Autodesk Fusion 360 part; units mm, degrees
(part 14 of 19)
  spline S154 degree 3 poles (24.0633, 11.8257) (24.3884, 11.9073) (24.7337, 11.9631) (25.4345, 12.0396) (25.8145, 12.0581) (26.1868, 12.059) knots -0.210627 -0.210627 -0.210627 -0.210627 -0.111696 -0.111696 0 0 0 0
  spline S155 degree 3 poles (23.9494, 11.8782) (23.9537, 11.8696) (23.9592, 11.8616) (23.9723, 11.8475) (23.9799, 11.8414) (23.9994, 11.8299) (24.0118, 11.8255) (24.0376, 11.8218) (24.0507, 11.8225) (24.0633, 11.8257) knots -0.013599 -0.013599 -0.013599 -0.013599 -0.010706 -0.010706 -0.007813 -0.007813 -0.003906 -0.003906 0 0 0 0
  arc A79 (23.9494, 11.8782) -> (23.6868, 12.3936) centre (0, 0) ccw
  spline S156 degree 3 poles (23.7112, 12.5167) (23.7038, 12.5105) (23.6974, 12.5033) (23.6867, 12.4872) (23.6826, 12.4784) (23.6759, 12.4568) (23.6746, 12.4437) (23.677, 12.4178) (23.6807, 12.4051) (23.6868, 12.3936) knots -0.013599 -0.013599 -0.013599 -0.013599 -0.010706 -0.010706 -0.007813 -0.007813 -0.003906 -0.003906 0 0 0 0
  spline S157 degree 3 poles (25.1482, 14.0975) (24.9286, 13.7968) (24.6903, 13.5003) (24.2164, 12.9783) (23.9684, 12.7317) (23.7112, 12.5167) knots -0.220678 -0.220678 -0.220678 -0.220678 -0.107909 -0.107909 -0.008028 -0.008028 -0.008028 -0.008028
  arc A80 (25.1482, 14.0975) -> (24.7828, 14.7302) centre (0, 0) ccw
  spline S158 degree 3 poles (22.6954, 14.2762) (23.0102, 14.3914) (23.3477, 14.4829) (24.0367, 14.6323) (24.4127, 14.6904) (24.7828, 14.7302) knots -0.210627 -0.210627 -0.210627 -0.210627 -0.111696 -0.111696 0 0 0 0
  spline S159 degree 3 poles (22.5766, 14.3165) (22.5817, 14.3084) (22.588, 14.301) (22.6026, 14.2884) (22.6107, 14.2831) (22.6313, 14.2737) (22.6441, 14.2707) (22.6702, 14.2697) (22.6831, 14.2717) (22.6954, 14.2762) knots -0.013599 -0.013599 -0.013599 -0.013599 -0.010706 -0.010706 -0.007813 -0.007813 -0.003906 -0.003906 0 0 0 0
  arc A81 (22.5766, 14.3165) -> (22.2615, 14.8017) centre (0, 0) ccw
  spline S160 degree 3 poles (22.273, 14.9266) (22.2663, 14.9197) (22.2606, 14.9118) (22.2517, 14.8947) (22.2485, 14.8856) (22.2441, 14.8633) (22.2442, 14.8502) (22.2493, 14.8246) (22.2543, 14.8125) (22.2615, 14.8017) knots -0.013599 -0.013599 -0.013599 -0.013599 -0.010706 -0.010706 -0.007813 -0.007813 -0.003906 -0.003906 0 0 0 0
  spline S161 degree 3 poles (23.5368, 16.6489) (23.3499, 16.327) (23.1439, 16.0071) (22.7272, 15.4385) (22.5063, 15.1674) (22.273, 14.9266) knots -0.220678 -0.220678 -0.220678 -0.220678 -0.107909 -0.107909 -0.008028 -0.008028 -0.008028 -0.008028
  arc A82 (23.5368, 16.6489) -> (23.1074, 17.24) centre (0, 0) ccw
  spline S162 degree 3 poles (21.0788, 16.5703) (21.3798, 16.7177) (21.7059, 16.8441) (22.3755, 17.0646) (22.7434, 17.1617) (23.1074, 17.24) knots -0.210627 -0.210627 -0.210627 -0.210627 -0.111696 -0.111696 0 0 0 0
  spline S163 degree 3 poles (20.9564, 16.598) (20.9624, 16.5904) (20.9694, 16.5838) (20.9852, 16.5727) (20.9939, 16.5683) (21.0154, 16.5611) (21.0284, 16.5594) (21.0544, 16.5612) (21.0671, 16.5645) (21.0788, 16.5703) knots -0.013599 -0.013599 -0.013599 -0.013599 -0.010706 -0.010706 -0.007813 -0.007813 -0.003906 -0.003906 0 0 0 0
  arc A83 (20.9564, 16.598) -> (20.5924, 17.0475) centre (0, 0) ccw
  spline S164 degree 3 poles (20.5907, 17.173) (20.5848, 17.1654) (20.5799, 17.157) (20.5728, 17.1391) (20.5706, 17.1296) (20.5686, 17.1071) (20.5701, 17.094) (20.5778, 17.0691) (20.5841, 17.0576) (20.5924, 17.0475) knots -0.013599 -0.013599 -0.013599 -0.013599 -0.010706 -0.010706 -0.007813 -0.007813 -0.003906 -0.003906 0 0 0 0
  spline S165 degree 3 poles (21.6676, 19.018) (21.5153, 18.6782) (21.3439, 18.3387) (20.9889, 17.7295) (20.7975, 17.4368) (20.5907, 17.173) knots -0.220678 -0.220678 -0.220678 -0.220678 -0.107909 -0.107909 -0.008028 -0.008028 -0.008028 -0.008028
  arc A84 (21.6676, 19.018) -> (21.1787, 19.561) centre (0, 0) ccw
  spline S166 degree 3 poles (19.2312, 18.6828) (19.5152, 18.861) (19.8263, 19.0207) (20.4692, 19.31) (20.8249, 19.445) (21.1787, 19.561) knots -0.210627 -0.210627 -0.210627 -0.210627 -0.111696 -0.111696 0 0 0 0
  spline S167 degree 3 poles (19.1066, 18.6976) (19.1134, 18.6907) (19.1211, 18.6848) (19.1379, 18.6755) (19.147, 18.672) (19.1691, 18.6671) (19.1823, 18.6668) (19.2079, 18.6712) (19.2202, 18.6759) (19.2312, 18.6828) knots -0.013599 -0.013599 -0.013599 -0.013599 -0.010706 -0.010706 -0.007813 -0.007813 -0.003906 -0.003906 0 0 0 0
  arc A85 (19.1066, 18.6976) -> (18.6976, 19.1066) centre (0, 0) ccw
  spline S168 degree 3 poles (18.6828, 19.2312) (18.6777, 19.2231) (18.6738, 19.2142) (18.6686, 19.1956) (18.6674, 19.186) (18.6678, 19.1633) (18.6706, 19.1505) (18.6809, 19.1266) (18.6883, 19.1157) (18.6976, 19.1066) knots -0.013599 -0.013599 -0.013599 -0.013599 -0.010706 -0.010706 -0.007813 -0.007813 -0.003906 -0.003906 0 0 0 0
  spline S169 degree 3 poles (19.561, 21.1787) (19.445, 20.8249) (19.31, 20.4692) (19.0207, 19.8263) (18.861, 19.5152) (18.6828, 19.2312) knots -0.220678 -0.220678 -0.220678 -0.220678 -0.107909 -0.107909 -0.008028 -0.008028 -0.008028 -0.008028
  arc A86 (19.561, 21.1787) -> (19.018, 21.6676) centre (0, 0) ccw
  spline S170 degree 3 poles (17.173, 20.5907) (17.4368, 20.7975) (17.7295, 20.9889) (18.3387, 21.3439) (18.6782, 21.5153) (19.018, 21.6676) knots -0.210627 -0.210627 -0.210627 -0.210627 -0.111696 -0.111696 0 0 0 0
  spline S171 degree 3 poles (17.0475, 20.5924) (17.055, 20.5862) (17.0632, 20.5812) (17.081, 20.5736) (17.0904, 20.5711) (17.1129, 20.5686) (17.126, 20.5696) (17.151, 20.5767) (17.1628, 20.5827) (17.173, 20.5907) knots -0.013599 -0.013599 -0.013599 -0.013599 -0.010706 -0.010706 -0.007813 -0.007813 -0.003906 -0.003906 0 0 0 0
  arc A87 (17.0475, 20.5924) -> (16.598, 20.9564) centre (0, 0) ccw
  spline S172 degree 3 poles (16.5703, 21.0788) (16.566, 21.0701) (16.5631, 21.0609) (16.5599, 21.0419) (16.5597, 21.0322) (16.5624, 21.0097) (16.5665, 20.9972) (16.5793, 20.9745) (16.5878, 20.9645) (16.598, 20.9564) knots -0.013599 -0.013599 -0.013599 -0.013599 -0.010706 -0.010706 -0.007813 -0.007813 -0.003906 -0.003906 0 0 0 0
  spline S173 degree 3 poles (17.24, 23.1074) (17.1617, 22.7434) (17.0646, 22.3755) (16.8441, 21.7059) (16.7177, 21.3798) (16.5703, 21.0788) knots -0.220678 -0.220678 -0.220678 -0.220678 -0.107909 -0.107909 -0.008028 -0.008028 -0.008028 -0.008028
  arc A88 (17.24, 23.1074) -> (16.6489, 23.5368) centre (0, 0) ccw
  spline S174 degree 3 poles (14.9266, 22.273) (15.1674, 22.5063) (15.4385, 22.7272) (16.0071, 23.1439) (16.327, 23.3499) (16.6489, 23.5368) knots -0.210627 -0.210627 -0.210627 -0.210627 -0.111696 -0.111696 0 0 0 0
  spline S175 degree 3 poles (14.8017, 22.2615) (14.8097, 22.2562) (14.8184, 22.252) (14.8369, 22.2464) (14.8465, 22.2449) (14.8691, 22.2447) (14.882, 22.2471) (14.9062, 22.2568) (14.9173, 22.2639) (14.9266, 22.273) knots -0.013599 -0.013599 -0.013599 -0.013599 -0.010706 -0.010706 -0.007813 -0.007813 -0.003906 -0.003906 0 0 0 0
  arc A89 (14.8017, 22.2615) -> (14.3165, 22.5766) centre (0, 0) ccw
  spline S176 degree 3 poles (14.2762, 22.6954) (14.2729, 22.6863) (14.2709, 22.6768) (14.2697, 22.6576) (14.2705, 22.6479) (14.2756, 22.6258) (14.2809, 22.6138) (14.296, 22.5926) (14.3055, 22.5835) (14.3165, 22.5766) knots -0.013599 -0.013599 -0.013599 -0.013599 -0.010706 -0.010706 -0.007813 -0.007813 -0.003906 -0.003906 0 0 0 0
  spline S177 degree 3 poles (14.7302, 24.7828) (14.6904, 24.4127) (14.6323, 24.0367) (14.4829, 23.3477) (14.3914, 23.0102) (14.2762, 22.6954) knots -0.220678 -0.220678 -0.220678 -0.220678 -0.107909 -0.107909 -0.008028 -0.008028 -0.008028 -0.008028
  arc A90 (14.7302, 24.7828) -> (14.0975, 25.1482) centre (0, 0) ccw
  spline S178 degree 3 poles (12.5167, 23.7112) (12.7317, 23.9684) (12.9783, 24.2164) (13.5003, 24.6903) (13.7968, 24.9286) (14.0975, 25.1482) knots -0.210627 -0.210627 -0.210627 -0.210627 -0.111696 -0.111696 0 0 0 0
  spline S179 degree 3 poles (12.3936, 23.6868) (12.4022, 23.6823) (12.4113, 23.6791) (12.4302, 23.6754) (12.4399, 23.6749) (12.4625, 23.6771) (12.4751, 23.6808) (12.4981, 23.693) (12.5083, 23.7012) (12.5167, 23.7112) knots -0.013599 -0.013599 -0.013599 -0.013599 -0.010706 -0.010706 -0.007813 -0.007813 -0.003906 -0.003906 0 0 0 0
  arc A91 (12.3936, 23.6868) -> (11.8782, 23.9494) centre (0, 0) ccw
  spline S180 degree 3 poles (11.8257, 24.0633) (11.8233, 24.054) (11.8223, 24.0443) (11.8231, 24.025) (11.8249, 24.0155) (11.8323, 23.9941) (11.8389, 23.9827) (11.8561, 23.9632) (11.8665, 23.9552) (11.8782, 23.9494) knots -0.013599 -0.013599 -0.013599 -0.013599 -0.010706 -0.010706 -0.007813 -0.007813 -0.003906 -0.003906 0 0 0 0
  spline S181 degree 3 poles (12.059, 26.1868) (12.0581, 25.8145) (12.0396, 25.4345) (11.9631, 24.7337) (11.9073, 24.3884) (11.8257, 24.0633) knots -0.220678 -0.220678 -0.220678 -0.220678 -0.107909 -0.107909 -0.008028 -0.008028 -0.008028 -0.008028
  arc A92 (12.059, 26.1868) -> (11.3915, 26.484) centre (0, 0) ccw
  spline S182 degree 3 poles (9.9696, 24.8897) (10.1566, 25.1679) (10.3759, 25.4404) (10.8455, 25.9662) (11.1155, 26.2342) (11.3915, 26.484) knots -0.210627 -0.210627 -0.210627 -0.210627 -0.111696 -0.111696 0 0 0 0
  spline S183 degree 3 poles (9.8498, 24.8525) (9.8587, 24.8489) (9.8682, 24.8467) (9.8874, 24.845) (9.8971, 24.8455) (9.9193, 24.85) (9.9314, 24.8551) (9.9531, 24.8696) (9.9624, 24.8789) (9.9696, 24.8897) knots -0.013599 -0.013599 -0.013599 -0.013599 -0.010706 -0.010706 -0.007813 -0.007813 -0.003906 -0.003906 0 0 0 0
  arc A93 (9.8498, 24.8525) -> (9.3097, 25.0598) centre (0, 0) ccw
  spline S184 degree 3 poles (9.2456, 25.1676) (9.2442, 25.1581) (9.2442, 25.1484) (9.2471, 25.1293) (9.2499, 25.12) (9.2594, 25.0995) (9.2672, 25.0888) (9.2863, 25.0712) (9.2975, 25.0643) (9.3097, 25.0598) knots -0.013599 -0.013599 -0.013599 -0.013599 -0.010706 -0.010706 -0.007813 -0.007813 -0.003906 -0.003906 0 0 0 0
  spline S185 degree 3 poles (9.2557, 27.3039) (9.2937, 26.9335) (9.315, 26.5537) (9.3122, 25.8487) (9.2928, 25.4995) (9.2456, 25.1676) knots -0.220678 -0.220678 -0.220678 -0.220678 -0.107909 -0.107909 -0.008028 -0.008028 -0.008028 -0.008028
  arc A94 (9.2557, 27.3039) -> (8.5608, 27.5296) centre (0, 0) ccw
  spline S186 degree 3 poles (7.3133, 25.7954) (7.4702, 26.0917) (7.6598, 26.3856) (8.0719, 26.9576) (8.3124, 27.2523) (8.5608, 27.5296) knots -0.210627 -0.210627 -0.210627 -0.210627 -0.111696 -0.111696 0 0 0 0
  spline S187 degree 3 poles (7.198, 25.7459) (7.2073, 25.7433) (7.2169, 25.7421) (7.2362, 25.7424) (7.2458, 25.7439) (7.2674, 25.7508) (7.2789, 25.757) (7.2989, 25.7737) (7.3072, 25.7839) (7.3133, 25.7954) knots -0.013599 -0.013599 -0.013599 -0.013599 -0.010706 -0.010706 -0.007813 -0.007813 -0.003906 -0.003906 0 0 0 0
  arc A95 (7.198, 25.7459) -> (6.6393, 25.8956) centre (0, 0) ccw
  spline S188 degree 3 poles (6.5642, 25.9962) (6.5638, 25.9865) (6.5649, 25.9769) (6.5697, 25.9582) (6.5734, 25.9493) (6.5851, 25.9298) (6.5939, 25.9201) (6.6148, 25.9045) (6.6267, 25.8989) (6.6393, 25.8956) knots -0.013599 -0.013599 -0.013599 -0.013599 -0.010706 -0.010706 -0.007813 -0.007813 -0.003906 -0.003906 0 0 0 0
  spline S189 degree 3 poles (6.351, 28.1218) (6.4275, 27.7574) (6.4884, 27.3819) (6.5592, 26.6805) (6.5765, 26.3312) (6.5642, 25.9962) knots -0.220678 -0.220678 -0.220678 -0.220678 -0.107909 -0.107909 -0.008028 -0.008028 -0.008028 -0.008028
  arc A96 (6.351, 28.1218) -> (5.6363, 28.2737) centre (0, 0) ccw
  spline S190 degree 3 poles (4.5769, 26.4186) (4.702, 26.7296) (4.8598, 27.0417) (5.2098, 27.6537) (5.4182, 27.9719) (5.6363, 28.2737) knots -0.210627 -0.210627 -0.210627 -0.210627 -0.111696 -0.111696 0 0 0 0
  spline S191 degree 3 poles (4.4674, 26.3573) (4.4769, 26.3557) (4.4866, 26.3554) (4.5058, 26.3578) (4.5151, 26.3603) (4.5359, 26.3693) (4.5467, 26.3768) (4.5649, 26.3955) (4.572, 26.4065) (4.5769, 26.4186) knots -0.013599 -0.013599 -0.013599 -0.013599 -0.010706 -0.010706 -0.007813 -0.007813 -0.003906 -0.003906 0 0 0 0
  arc A97 (4.4674, 26.3573) -> (3.8961, 26.4478) centre (0, 0) ccw
  spline S192 degree 3 poles (3.8109, 26.5399) (3.8115, 26.5303) (3.8136, 26.5208) (3.8203, 26.5027) (3.825, 26.4942) (3.8386, 26.4761) (3.8484, 26.4674) (3.8708, 26.4541) (3.8832, 26.4497) (3.8961, 26.4478) knots -0.013599 -0.013599 -0.013599 -0.013599 -0.010706 -0.010706 -0.007813 -0.007813 -0.003906 -0.003906 0 0 0 0
  spline S193 degree 3 poles (3.3766, 28.6316) (3.4908, 28.2772) (3.5906, 27.9101) (3.7344, 27.2199) (3.7881, 26.8744) (3.8109, 26.5399) knots -0.220678 -0.220678 -0.220678 -0.220678 -0.107909 -0.107909 -0.008028 -0.008028 -0.008028 -0.008028
  arc A98 (3.3766, 28.6316) -> (2.65, 28.708) centre (0, 0) ccw
  spline S194 degree 3 poles (1.7903, 26.7523) (1.8822, 27.0747) (2.0065, 27.4015) (2.2907, 28.0467) (2.4646, 28.385) (2.65, 28.708) knots -0.210627 -0.210627 -0.210627 -0.210627 -0.111696 -0.111696 0 0 0 0
  spline S195 degree 3 poles (1.6879, 26.6799) (1.6975, 26.6793) (1.7071, 26.68) (1.7259, 26.6844) (1.735, 26.6879) (1.7547, 26.699) (1.7647, 26.7076) (1.7808, 26.728) (1.7868, 26.7397) (1.7903, 26.7523) knots -0.013599 -0.013599 -0.013599 -0.013599 -0.010706 -0.010706 -0.007813 -0.007813 -0.003906 -0.003906 0 0 0 0
  arc A99 (1.6879, 26.6799) -> (1.1102, 26.7101) centre (0, 0) ccw
  spline S196 degree 3 poles (1.0158, 26.7929) (1.0175, 26.7834) (1.0205, 26.7741) (1.0291, 26.7569) (1.0346, 26.7489) (1.0501, 26.7323) (1.0607, 26.7246) (1.0844, 26.7138) (1.0972, 26.7107) (1.1102, 26.7101) knots -0.013599 -0.013599 -0.013599 -0.013599 -0.010706 -0.010706 -0.007813 -0.007813 -0.003906 -0.003906 0 0 0 0
  spline S197 degree 3 poles (0.3653, 28.8277) (0.5159, 28.4872) (0.6536, 28.1325) (0.8687, 27.4612) (0.9582, 27.1231) (1.0158, 26.7929) knots -0.220678 -0.220678 -0.220678 -0.220678 -0.107909 -0.107909 -0.008028 -0.008028 -0.008028 -0.008028
  arc A100 (0.3653, 28.8277) -> (-0.3653, 28.8277) centre (0, 0) ccw
  spline S198 degree 3 poles (-1.0158, 26.7929) (-0.9582, 27.1231) (-0.8687, 27.4612) (-0.6536, 28.1325) (-0.5159, 28.4872) (-0.3653, 28.8277) knots -0.210627 -0.210627 -0.210627 -0.210627 -0.111696 -0.111696 0 0 0 0
  spline S199 degree 3 poles (-1.1102, 26.7101) (-1.1006, 26.7105) (-1.091, 26.7123) (-1.0728, 26.7186) (-1.0642, 26.723) (-1.0457, 26.7362) (-1.0367, 26.7457) (-1.0228, 26.7678) (-1.0181, 26.78) (-1.0158, 26.7929) knots -0.013599 -0.013599 -0.013599 -0.013599 -0.010706 -0.010706 -0.007813 -0.007813 -0.003906 -0.003906 0 0 0 0
  arc A101 (-1.1102, 26.7101) -> (-1.6879, 26.6799) centre (0, 0) ccw
  spline S200 degree 3 poles (-1.7903, 26.7523) (-1.7877, 26.743) (-1.7837, 26.7341) (-1.7734, 26.7179) (-1.7671, 26.7105) (-1.75, 26.6957) (-1.7386, 26.6891) (-1.7139, 26.6808) (-1.7008, 26.679) (-1.6879, 26.6799) knots -0.013599 -0.013599 -0.013599 -0.013599 -0.010706 -0.010706 -0.007813 -0.007813 -0.003906 -0.003906 0 0 0 0
  spline S201 degree 3 poles (-2.65, 28.708) (-2.4646, 28.385) (-2.2907, 28.0467) (-2.0065, 27.4015) (-1.8822, 27.0747) (-1.7903, 26.7523) knots -0.220678 -0.220678 -0.220678 -0.220678 -0.107909 -0.107909 -0.008028 -0.008028 -0.008028 -0.008028
  arc A102 (-2.65, 28.708) -> (-3.3766, 28.6316) centre (0, 0) ccw
  spline S202 degree 3 poles (-3.8109, 26.5399) (-3.7881, 26.8744) (-3.7344, 27.2199) (-3.5906, 27.9101) (-3.4908, 28.2772) (-3.3766, 28.6316) knots -0.210627 -0.210627 -0.210627 -0.210627 -0.111696 -0.111696 0 0 0 0
  spline S203 degree 3 poles (-3.8961, 26.4478) (-3.8865, 26.4492) (-3.8773, 26.452) (-3.8598, 26.4601) (-3.8517, 26.4654) (-3.8347, 26.4804) (-3.8267, 26.4908) (-3.8152, 26.5142) (-3.8118, 26.5269) (-3.8109, 26.5399) knots -0.013599 -0.013599 -0.013599 -0.013599 -0.010706 -0.010706 -0.007813 -0.007813 -0.003906 -0.003906 0 0 0 0
  arc A103 (-3.8961, 26.4478) -> (-4.4674, 26.3573) centre (0, 0) ccw
  spline S204 degree 3 poles (-4.5769, 26.4186) (-4.5733, 26.4096) (-4.5684, 26.4012) (-4.5564, 26.3861) (-4.5494, 26.3795) (-4.5308, 26.3665) (-4.5188, 26.3612) (-4.4934, 26.3555) (-4.4803, 26.3551) (-4.4674, 26.3573) knots -0.013599 -0.013599 -0.013599 -0.013599 -0.010706 -0.010706 -0.007813 -0.007813 -0.003906 -0.003906 0 0 0 0
  spline S205 degree 3 poles (-5.6363, 28.2737) (-5.4182, 27.9719) (-5.2098, 27.6537) (-4.8598, 27.0417) (-4.702, 26.7296) (-4.5769, 26.4186) knots -0.220678 -0.220678 -0.220678 -0.220678 -0.107909 -0.107909 -0.008028 -0.008028 -0.008028 -0.008028
  arc A104 (-5.6363, 28.2737) -> (-6.351, 28.1218) centre (0, 0) ccw
  spline S206 degree 3 poles (-6.5642, 25.9962) (-6.5765, 26.3312) (-6.5592, 26.6805) (-6.4884, 27.3819) (-6.4275, 27.7574) (-6.351, 28.1218) knots -0.210627 -0.210627 -0.210627 -0.210627 -0.111696 -0.111696 0 0 0 0
  spline S207 degree 3 poles (-6.6393, 25.8956) (-6.6299, 25.898) (-6.621, 25.9018) (-6.6045, 25.9117) (-6.5969, 25.9178) (-6.5816, 25.9345) (-6.5748, 25.9457) (-6.5658, 25.9702) (-6.5637, 25.9831) (-6.5642, 25.9962) knots -0.013599 -0.013599 -0.013599 -0.013599 -0.010706 -0.010706 -0.007813 -0.007813 -0.003906 -0.003906 0 0 0 0
  arc A105 (-6.6393, 25.8956) -> (-7.198, 25.7459) centre (0, 0) ccw
  spline S208 degree 3 poles (-7.3133, 25.7954) (-7.3088, 25.7869) (-7.3031, 25.7791) (-7.2896, 25.7653) (-7.2819, 25.7594) (-7.2621, 25.7485) (-7.2495, 25.7444) (-7.2237, 25.7414) (-7.2106, 25.7424) (-7.198, 25.7459) knots -0.013599 -0.013599 -0.013599 -0.013599 -0.010706 -0.010706 -0.007813 -0.007813 -0.003906 -0.003906 0 0 0 0
  spline S209 degree 3 poles (-8.5608, 27.5296) (-8.3124, 27.2523) (-8.0719, 26.9576) (-7.6598, 26.3856) (-7.4702, 26.0917) (-7.3133, 25.7954) knots -0.220678 -0.220678 -0.220678 -0.220678 -0.107909 -0.107909 -0.008028 -0.008028 -0.008028 -0.008028
  arc A106 (-8.5608, 27.5296) -> (-9.2557, 27.3039) centre (0, 0) ccw
  spline S210 degree 3 poles (-9.2456, 25.1676) (-9.2928, 25.4995) (-9.3122, 25.8487) (-9.315, 26.5537) (-9.2937, 26.9335) (-9.2557, 27.3039) knots -0.210627 -0.210627 -0.210627 -0.210627 -0.111696 -0.111696 0 0 0 0
  spline S211 degree 3 poles (-9.3097, 25.0598) (-9.3007, 25.0631) (-9.2922, 25.0678) (-9.2768, 25.0794) (-9.27, 25.0863) (-9.2565, 25.1045) (-9.2508, 25.1163) (-9.2444, 25.1416) (-9.2437, 25.1547) (-9.2456, 25.1676) knots -0.013599 -0.013599 -0.013599 -0.013599 -0.010706 -0.010706 -0.007813 -0.007813 -0.003906 -0.003906 0 0 0 0
  arc A107 (-9.3097, 25.0598) -> (-9.8498, 24.8525) centre (0, 0) ccw
  spline S212 degree 3 poles (-9.9696, 24.8897) (-9.9642, 24.8817) (-9.9577, 24.8745) (-9.9429, 24.8622) (-9.9346, 24.8572) (-9.9137, 24.8483) (-9.9008, 24.8456) (-9.8748, 24.8453) (-9.8619, 24.8477) (-9.8498, 24.8525) knots -0.013599 -0.013599 -0.013599 -0.013599 -0.010706 -0.010706 -0.007813 -0.007813 -0.003906 -0.003906 0 0 0 0
  spline S213 degree 3 poles (-11.3915, 26.484) (-11.1155, 26.2342) (-10.8455, 25.9662) (-10.3759, 25.4404) (-10.1566, 25.1679) (-9.9696, 24.8897) knots -0.220678 -0.220678 -0.220678 -0.220678 -0.107909 -0.107909 -0.008028 -0.008028 -0.008028 -0.008028
  arc A108 (-11.3915, 26.484) -> (-12.059, 26.1868) centre (0, 0) ccw
  spline S214 degree 3 poles (-11.8257, 24.0633) (-11.9073, 24.3884) (-11.9631, 24.7337) (-12.0396, 25.4345) (-12.0581, 25.8145) (-12.059, 26.1868) knots -0.210627 -0.210627 -0.210627 -0.210627 -0.111696 -0.111696 0 0 0 0
  spline S215 degree 3 poles (-11.8782, 23.9494) (-11.8696, 23.9537) (-11.8616, 23.9592) (-11.8475, 23.9723) (-11.8414, 23.9799) (-11.8299, 23.9994) (-11.8255, 24.0118) (-11.8218, 24.0376) (-11.8225, 24.0507) (-11.8257, 24.0633) knots -0.013599 -0.013599 -0.013599 -0.013599 -0.010706 -0.010706 -0.007813 -0.007813 -0.003906 -0.003906 0 0 0 0
  arc A109 (-11.8782, 23.9494) -> (-12.1366, 23.8195) centre (0, 0) ccw
  circle A110 centre (0, 0) radius 8
  circle A111 centre (0, 0) radius 10
  circle A112 centre (0, 0) radius 25
  line L2 (0, -40) -> (0, 0)
  line L3 (34.641, -20) -> (0, 0)
  line L4 (34.641, 20) -> (0, 0)
  line L5 (0, 40) -> (0, 0)
  line L6 (-34.641, 20) -> (0, 0)
  line L7 (-34.641, -20) -> (0, 0)
  dimension "d73" = 20
  dimension "d75" = 360
  constraint coincident A0.centre A1.centre
  constraint vertical L2
  measures "d73" diameter of A111
extrude "Estrusione9" cut sketch "Schizzo7" against normal blind 1 contours A0 A111 A112 L5 L6 | A111 A112 L3 L4 | A111 A112 L2 L7 in component "Spur Gear (60 teeth) (1)"
sketch "Schizzo9" plane through (0, 0, 2) normal (0, 0, 1) x (-1, 0, 0)
  line L0 (8.6603, -5) -> (21.6506, -12.5)
  arc A0 (21.6506, -12.5) -> (21.6506, 12.5) centre (0, 0) ccw
  line L1 (21.6506, 12.5) -> (8.6603, 5)
  arc A1 (8.6603, -5) -> (8.6603, 5) centre (0, 0) ccw
  line L2 (7.9146, 3.8207) -> (7.9146, -14.1793) construction
  line L3 (7.9146, -14.1793) -> (20.9146, -14.1793) construction
  line L4 (20.9146, -14.1793) -> (20.9146, 3.8207) construction
  line L5 (20.9146, 3.8207) -> (7.9146, 3.8207) construction
  dimension "d78" = 5
  text T0 "2h" font "Arial" height 5 bold align left top in box 18 x 13 at (7.9146, 3.8207) x (0, -1) y (1, 0) spacing 1 kerned
extrude "Estrusione10" add sketch "Schizzo9" along normal blind 1 text T0 in component "Spur Gear (60 teeth) (1)"
component "Spur Gear (60 teeth) (1)" placed x (1, 0, 0) y (0, 1, 0) z (0, 0, 1) at (0, 0, 0)

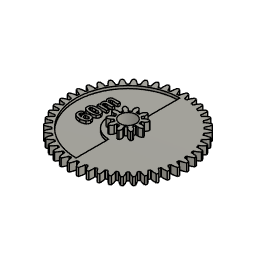
design "6 intermedio ore"
description: Spur Gear; Module: 1.000000; Num Teeth: 44; Pressure Angle: 20.000000; Backlash: 0.00 mm
description: Spur Gear; Module: 1.000000; Num Teeth: 10; Pressure Angle: 20.000000; Backlash: 0.00 mm
Autodesk Fusion 360 part; units mm, degrees
sketch "Schizzo1" plane through (0, 0, 0) normal (0, 0, 1) x (1, 0, 0) in component "Spur Gear (44 teeth)"
  circle A0 centre (0, 0) radius 20.7492
  circle A1 centre (0, 0) radius 3.1
extrude "Estrusione1" add sketch "Schizzo1" along normal blind 3 makes body 1 in component "Spur Gear (44 teeth)"
sketch "Schizzo2" plane through (0, 0, 0) normal (0, 0, 1) x (1, 0, 0) in component "Spur Gear (44 teeth)"
  spline S0 degree 5 poles (20.6468, -1.0457) (20.6535, -1.0457) (20.667, -1.0458) (20.6873, -1.0456) (20.7143, -1.0451) (20.7481, -1.044) (20.7819, -1.0422) (20.8157, -1.04) (20.8495, -1.0372) (20.8833, -1.034) (20.9172, -1.0304) (20.951, -1.0264) (20.9848, -1.022) (21.0187, -1.0174) (21.0525, -1.0125) (21.0863, -1.0073) (21.1202, -1.0019) (21.154, -0.9961) (21.1878, -0.9902) (21.2216, -0.9839) (21.2554, -0.9774) (21.2892, -0.9707) (21.323, -0.9637) (21.3568, -0.9565) (21.3906, -0.9491) (21.4244, -0.9415) (21.4581, -0.9337) (21.4919, -0.9256) (21.5256, -0.9174) (21.5594, -0.9089) (21.5931, -0.9002) (21.6268, -0.8914) (21.6605, -0.8823) (21.6942, -0.8731) (21.7279, -0.8636) (21.7616, -0.854) (21.7952, -0.8442) (21.8289, -0.8343) (21.8625, -0.8241) (21.8961, -0.8138) (21.9298, -0.8033) (21.9634, -0.7926) (21.9969, -0.7817) (22.0305, -0.7707) (22.0641, -0.7595) (22.0976, -0.7481) (22.1311, -0.7366) (22.1646, -0.7249) (22.1981, -0.7131) (22.2316, -0.7011) (22.2651, -0.6889) (22.2985, -0.6766) (22.332, -0.6642) (22.3654, -0.6515) (22.3988, -0.6387) (22.4322, -0.6258) (22.4655, -0.6127) (22.4989, -0.5995) (22.5322, -0.5861) (22.5655, -0.5726) (22.5988, -0.5589) (22.6321, -0.5451) (22.6653, -0.5311) (22.6986, -0.517) (22.7318, -0.5027) (22.765, -0.4883) (22.7982, -0.4738) (22.8313, -0.4591) (22.8645, -0.4443) (22.8976, -0.4294) (22.9307, -0.4143) (22.9571, -0.4021) (22.977, -0.3929) (22.9902, -0.3867) (22.9968, -0.3836) knots 0 0 0 0 0 0 0.01428571 0.02857143 0.04285714 0.05714286 0.07142857 0.08571429 0.1 0.11428571 0.12857143 0.14285714 0.15714286 0.17142857 0.18571429 0.2 0.21428571 0.22857143 0.24285714 0.25714286 0.27142857 0.28571429 0.3 0.31428571 0.32857143 0.34285714 0.35714286 0.37142857 0.38571429 0.4 0.41428571 0.42857143 0.44285714 0.45714286 0.47142857 0.48571429 0.5 0.51428571 0.52857143 0.54285714 0.55714286 0.57142857 0.58571429 0.6 0.61428571 0.62857143 0.64285714 0.65714286 0.67142857 0.68571429 0.7 0.71428571 0.72857143 0.74285714 0.75714286 0.77142857 0.78571429 0.8 0.81428571 0.82857143 0.84285714 0.85714286 0.87142857 0.88571429 0.9 0.91428571 0.92857143 0.94285714 0.95714286 0.97142857 0.98571429 1 1 1 1 1 1
  spline S1 degree 5 poles (20.6468, 1.0457) (20.6535, 1.0457) (20.667, 1.0458) (20.6873, 1.0456) (20.7143, 1.0451) (20.7481, 1.044) (20.7819, 1.0422) (20.8157, 1.04) (20.8495, 1.0372) (20.8833, 1.034) (20.9172, 1.0304) (20.951, 1.0264) (20.9848, 1.022) (21.0187, 1.0174) (21.0525, 1.0125) (21.0863, 1.0073) (21.1202, 1.0019) (21.154, 0.9961) (21.1878, 0.9902) (21.2216, 0.9839) (21.2554, 0.9774) (21.2892, 0.9707) (21.323, 0.9637) (21.3568, 0.9565) (21.3906, 0.9491) (21.4244, 0.9415) (21.4581, 0.9337) (21.4919, 0.9256) (21.5256, 0.9174) (21.5594, 0.9089) (21.5931, 0.9002) (21.6268, 0.8914) (21.6605, 0.8823) (21.6942, 0.8731) (21.7279, 0.8636) (21.7616, 0.854) (21.7952, 0.8442) (21.8289, 0.8343) (21.8625, 0.8241) (21.8961, 0.8138) (21.9298, 0.8033) (21.9634, 0.7926) (21.9969, 0.7817) (22.0305, 0.7707) (22.0641, 0.7595) (22.0976, 0.7481) (22.1311, 0.7366) (22.1646, 0.7249) (22.1981, 0.7131) (22.2316, 0.7011) (22.2651, 0.6889) (22.2985, 0.6766) (22.332, 0.6642) (22.3654, 0.6515) (22.3988, 0.6387) (22.4322, 0.6258) (22.4655, 0.6127) (22.4989, 0.5995) (22.5322, 0.5861) (22.5655, 0.5726) (22.5988, 0.5589) (22.6321, 0.5451) (22.6653, 0.5311) (22.6986, 0.517) (22.7318, 0.5027) (22.765, 0.4883) (22.7982, 0.4738) (22.8313, 0.4591) (22.8645, 0.4443) (22.8976, 0.4294) (22.9307, 0.4143) (22.9571, 0.4021) (22.977, 0.3929) (22.9902, 0.3867) (22.9968, 0.3836) knots 0 0 0 0 0 0 0.01428571 0.02857143 0.04285714 0.05714286 0.07142857 0.08571429 0.1 0.11428571 0.12857143 0.14285714 0.15714286 0.17142857 0.18571429 0.2 0.21428571 0.22857143 0.24285714 0.25714286 0.27142857 0.28571429 0.3 0.31428571 0.32857143 0.34285714 0.35714286 0.37142857 0.38571429 0.4 0.41428571 0.42857143 0.44285714 0.45714286 0.47142857 0.48571429 0.5 0.51428571 0.52857143 0.54285714 0.55714286 0.57142857 0.58571429 0.6 0.61428571 0.62857143 0.64285714 0.65714286 0.67142857 0.68571429 0.7 0.71428571 0.72857143 0.74285714 0.75714286 0.77142857 0.78571429 0.8 0.81428571 0.82857143 0.84285714 0.85714286 0.87142857 0.88571429 0.9 0.91428571 0.92857143 0.94285714 0.95714286 0.97142857 0.98571429 1 1 1 1 1 1
  arc A0 (22.9968, -0.3836) -> (22.9968, 0.3836) centre (0, 0) ccw
  line L0 (20.6468, 1.0457) -> (20.6468, -1.0457)
  point P0 (20.8135, -1.04)
  point P1 (20.9807, -1.0225)
  point P2 (21.1483, -0.9971)
  point P3 (21.3162, -0.9651)
  point P4 (21.4842, -0.9274)
  point P5 (21.6524, -0.8845)
  point P6 (21.8206, -0.8367)
  point P7 (21.9888, -0.7843)
  point P8 (22.1571, -0.7276)
  point P9 (22.3253, -0.6666)
  point P10 (22.4934, -0.6017)
  point P11 (22.6613, -0.5328)
  point P12 (22.8292, -0.4601)
  point P13 (20.8135, 1.04)
  point P14 (20.9807, 1.0225)
  point P15 (21.1483, 0.9971)
  point P16 (21.3162, 0.9651)
  point P17 (21.4842, 0.9274)
  point P18 (21.6524, 0.8845)
  point P19 (21.8206, 0.8367)
  point P20 (21.9888, 0.7843)
  point P21 (22.1571, 0.7276)
  point P22 (22.3253, 0.6666)
  point P23 (22.4934, 0.6017)
  point P24 (22.6613, 0.5328)
  point P25 (22.8292, 0.4601)
extrude "Estrusione2" add sketch "Schizzo2" along normal blind 3 bodies 1 in component "Spur Gear (44 teeth)"
fillet "Raccordo1" radius 0.1 2 edges at (20.7229, 1.0448, 1.5) (20.7229, -1.0448, 1.5) on bodies 1 in component "Spur Gear (44 teeth)"
pattern_circular "Serie C1" count 44 over 360 about axis through (0, 0, 0) along (0, 0, 1) of "Estrusione2", "Raccordo1" in component "Spur Gear (44 teeth)"
sketch "Schizzo3" plane through (0, 0, 0) normal (0, 0, 1) x (1, 0, 0) in component "Spur Gear (44 teeth)"
  circle A0 centre (0, 0) radius 22 construction
sketch "Schizzo1 (2)" plane through (0, 0, 0) normal (0, 0, 1) x (1, 0, 0) in component "Spur Gear (10 teeth)"
  circle A0 centre (0, 0) radius 3.7492
  circle A1 centre (0, 0) radius 3.1
extrude "Estrusione1'" add sketch "Schizzo1 (2)" along normal blind 6 separate body makes body 2 in component "Spur Gear (10 teeth)"
sketch "Schizzo2 (2)" plane through (0, 0, 0) normal (0, 0, 1) x (1, 0, 0) in component "Spur Gear (10 teeth)"
  spline S0 degree 5 poles (4.6291, -0.8041) (4.6329, -0.8047) (4.6405, -0.8059) (4.6519, -0.8073) (4.6672, -0.8084) (4.6864, -0.8088) (4.7057, -0.8085) (4.7251, -0.8077) (4.7445, -0.8066) (4.7639, -0.8054) (4.7834, -0.804) (4.8029, -0.8024) (4.8224, -0.8004) (4.842, -0.7981) (4.8616, -0.7954) (4.8812, -0.7924) (4.9009, -0.7891) (4.9205, -0.7856) (4.9402, -0.7818) (4.9599, -0.7778) (4.9796, -0.7737) (4.9993, -0.7693) (5.019, -0.7646) (5.0388, -0.7598) (5.0585, -0.7547) (5.0783, -0.7493) (5.098, -0.7438) (5.1178, -0.738) (5.1375, -0.7321) (5.1573, -0.7259) (5.177, -0.7196) (5.1968, -0.7131) (5.2165, -0.7063) (5.2363, -0.6994) (5.256, -0.6923) (5.2757, -0.685) (5.2955, -0.6775) (5.3152, -0.6698) (5.3349, -0.6619) (5.3546, -0.6538) (5.3743, -0.6456) (5.394, -0.6372) (5.4136, -0.6286) (5.4333, -0.6198) (5.4529, -0.6109) (5.4725, -0.6018) (5.4921, -0.5925) (5.5117, -0.583) (5.5312, -0.5734) (5.5508, -0.5636) (5.5703, -0.5536) (5.5898, -0.5435) (5.6093, -0.5332) (5.6287, -0.5228) (5.6482, -0.5121) (5.6676, -0.5013) (5.6869, -0.4904) (5.7063, -0.4793) (5.7256, -0.468) (5.7449, -0.4566) (5.7642, -0.445) (5.7834, -0.4332) (5.8026, -0.4213) (5.8218, -0.4093) (5.8409, -0.397) (5.86, -0.3847) (5.8791, -0.3721) (5.8982, -0.3595) (5.9172, -0.3466) (5.9361, -0.3336) (5.9551, -0.3205) (5.9702, -0.3099) (5.9815, -0.3018) (5.989, -0.2964) (5.9928, -0.2937) knots 0 0 0 0 0 0 0.01428571 0.02857143 0.04285714 0.05714286 0.07142857 0.08571429 0.1 0.11428571 0.12857143 0.14285714 0.15714286 0.17142857 0.18571429 0.2 0.21428571 0.22857143 0.24285714 0.25714286 0.27142857 0.28571429 0.3 0.31428571 0.32857143 0.34285714 0.35714286 0.37142857 0.38571429 0.4 0.41428571 0.42857143 0.44285714 0.45714286 0.47142857 0.48571429 0.5 0.51428571 0.52857143 0.54285714 0.55714286 0.57142857 0.58571429 0.6 0.61428571 0.62857143 0.64285714 0.65714286 0.67142857 0.68571429 0.7 0.71428571 0.72857143 0.74285714 0.75714286 0.77142857 0.78571429 0.8 0.81428571 0.82857143 0.84285714 0.85714286 0.87142857 0.88571429 0.9 0.91428571 0.92857143 0.94285714 0.95714286 0.97142857 0.98571429 1 1 1 1 1 1
  spline S1 degree 5 poles (4.6291, 0.8041) (4.6329, 0.8047) (4.6405, 0.8059) (4.6519, 0.8073) (4.6672, 0.8084) (4.6864, 0.8088) (4.7057, 0.8085) (4.7251, 0.8077) (4.7445, 0.8066) (4.7639, 0.8054) (4.7834, 0.804) (4.8029, 0.8024) (4.8224, 0.8004) (4.842, 0.7981) (4.8616, 0.7954) (4.8812, 0.7924) (4.9009, 0.7891) (4.9205, 0.7856) (4.9402, 0.7818) (4.9599, 0.7778) (4.9796, 0.7737) (4.9993, 0.7693) (5.019, 0.7646) (5.0388, 0.7598) (5.0585, 0.7547) (5.0783, 0.7493) (5.098, 0.7438) (5.1178, 0.738) (5.1375, 0.7321) (5.1573, 0.7259) (5.177, 0.7196) (5.1968, 0.7131) (5.2165, 0.7063) (5.2363, 0.6994) (5.256, 0.6923) (5.2757, 0.685) (5.2955, 0.6775) (5.3152, 0.6698) (5.3349, 0.6619) (5.3546, 0.6538) (5.3743, 0.6456) (5.394, 0.6372) (5.4136, 0.6286) (5.4333, 0.6198) (5.4529, 0.6109) (5.4725, 0.6018) (5.4921, 0.5925) (5.5117, 0.583) (5.5312, 0.5734) (5.5508, 0.5636) (5.5703, 0.5536) (5.5898, 0.5435) (5.6093, 0.5332) (5.6287, 0.5228) (5.6482, 0.5121) (5.6676, 0.5013) (5.6869, 0.4904) (5.7063, 0.4793) (5.7256, 0.468) (5.7449, 0.4566) (5.7642, 0.445) (5.7834, 0.4332) (5.8026, 0.4213) (5.8218, 0.4093) (5.8409, 0.397) (5.86, 0.3847) (5.8791, 0.3721) (5.8982, 0.3595) (5.9172, 0.3466) (5.9361, 0.3336) (5.9551, 0.3205) (5.9702, 0.3099) (5.9815, 0.3018) (5.989, 0.2964) (5.9928, 0.2937) knots 0 0 0 0 0 0 0.01428571 0.02857143 0.04285714 0.05714286 0.07142857 0.08571429 0.1 0.11428571 0.12857143 0.14285714 0.15714286 0.17142857 0.18571429 0.2 0.21428571 0.22857143 0.24285714 0.25714286 0.27142857 0.28571429 0.3 0.31428571 0.32857143 0.34285714 0.35714286 0.37142857 0.38571429 0.4 0.41428571 0.42857143 0.44285714 0.45714286 0.47142857 0.48571429 0.5 0.51428571 0.52857143 0.54285714 0.55714286 0.57142857 0.58571429 0.6 0.61428571 0.62857143 0.64285714 0.65714286 0.67142857 0.68571429 0.7 0.71428571 0.72857143 0.74285714 0.75714286 0.77142857 0.78571429 0.8 0.81428571 0.82857143 0.84285714 0.85714286 0.87142857 0.88571429 0.9 0.91428571 0.92857143 0.94285714 0.95714286 0.97142857 0.98571429 1 1 1 1 1 1
  arc A0 (5.9928, -0.2937) -> (5.9928, 0.2937) centre (0, 0) ccw
  line L0 (3.684, -0.6416) -> (4.6291, -0.8041)
  line L1 (3.684, 0.6416) -> (4.6291, 0.8041)
  line L2 (3.684, -0.6416) -> (3.684, 0.6416)
  point P0 (4.7229, -0.8077)
  point P1 (4.8183, -0.8008)
  point P2 (4.9148, -0.7866)
  point P3 (5.0121, -0.7662)
  point P4 (5.11, -0.7403)
  point P5 (5.2082, -0.7091)
  point P6 (5.3067, -0.673)
  point P7 (5.4054, -0.6322)
  point P8 (5.504, -0.5867)
  point P9 (5.6025, -0.5368)
  point P10 (5.7007, -0.4824)
  point P11 (5.7986, -0.4238)
  point P12 (5.896, -0.3609)
  point P13 (4.7229, 0.8077)
  point P14 (4.8183, 0.8008)
  point P15 (4.9148, 0.7866)
  point P16 (5.0121, 0.7662)
  point P17 (5.11, 0.7403)
  point P18 (5.2082, 0.7091)
  point P19 (5.3067, 0.673)
  point P20 (5.4054, 0.6322)
  point P21 (5.504, 0.5867)
  point P22 (5.6025, 0.5368)
  point P23 (5.7007, 0.4824)
  point P24 (5.7986, 0.4238)
  point P25 (5.896, 0.3609)
extrude "Estrusione2'" add sketch "Schizzo2 (2)" along normal blind 6 bodies 2 in component "Spur Gear (10 teeth)"
fillet "Raccordo1'" radius 0.1 2 edges at (3.6936, -0.6433, 3) (3.6936, 0.6433, 3) on bodies 2 in component "Spur Gear (10 teeth)"
pattern_circular "Serie C1'" count 10 over 360 about axis through (0, 0, 0) along (0, 0, 1) of "Estrusione2'", "Raccordo1'" in component "Spur Gear (10 teeth)"
sketch "Schizzo3 (2)" plane through (0, 0, 0) normal (0, 0, 1) x (1, 0, 0) in component "Spur Gear (10 teeth)"
  circle A0 centre (0, 0) radius 5 construction
combine "Combina1" operation add target body 1 tool bodies 2 in component "Spur Gear (44 teeth)"